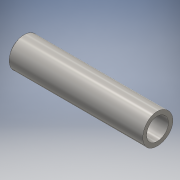
# Autodesk Inventor part: Nozzle 1 in drain
Saved by Autodesk Inventor 2016 (Build 200138000, 138)
## iProperties
Created: 2018-11-07
Part Number: Nozzle 1 in drain
Material: Steel, Alloy
Document SubType Name: Modeling
Designer: Wijaya
Mass: 476.569 g
Surface Area: 279.09 cm^2
Volume: 61.6519 cm^3
Density: 7.73 g/cm^3
Appearance: Semi-Polished
Author: Wijaya
Autodesk Inventor part; units mm, degrees
ref_plane "YZ Plane" through (0, 0, 0) normal (1, 0, 0) x (0, 1, 0)
ref_plane "XZ Plane" through (0, 0, 0) normal (0, 1, 0) x (-1, 0, 0)
ref_plane "XY Plane" through (0, 0, 0) normal (0, 0, 1) x (1, 0, 0)
sketch "Sketch2" plane through (0, 0, 0) normal (0, 0, 1) x (1, 0, 0)
  circle A0 centre (327.8, 0) radius 177.8
  point P0 (0, 0)
  dimension "d12" = 355.6
  dimension "d13" = 327.8
  constraints: 1 centre point, 1 horizontal alignment
  measures "d12" diameter of A0
  measures "d13" distance of point (0, 0) A0.centre
sketch "Sketch1" plane through (0, 0, 0) normal (0, 0, 1) x (1, 0, 0)
  line L0 (0, 0) -> (304, 0)
  line L1 (0, 13.75) -> (2.2636, 16.7)
  line L2 (2.2636, 16.7) -> (150.786, 16.7)
  line L3 (150.786, 16.7) -> (150.786, 12.15)
  line L4 (150.786, 12.15) -> (0, 12.15)
  circle A0 centre (327.8, 0) radius 177.8 projected
  line L5 (0, 13.75) -> (0, 12.15)
  dimension "d1" = 33.4
  dimension "d2" = 24.3
  dimension "d4" = 1.6
  dimension "d27" = 37.5
  constraints: 12 end point, 3 perpendicular, 1 horizontal, 1 parallel, 1 vertical alignment, 2 other
  measures "d1" diameter of L2 L0
  measures "d2" diameter of L4 L0
  measures "d4" distance from line of L4 L1.start
  measures "d27" angle of L5 L1
revolve "Revolution1" add sketch "Sketch1" angle 360 about axis through (0, 0, 0) along (1, 0, 0) picked at (150.7405, 14.6781) contours L1 L2 A0 L4 L5 | L3 L4 A0
extrude "Extrusion1" cut sketch "Sketch2" along normal mid plane 33.4
body "Solid1"
